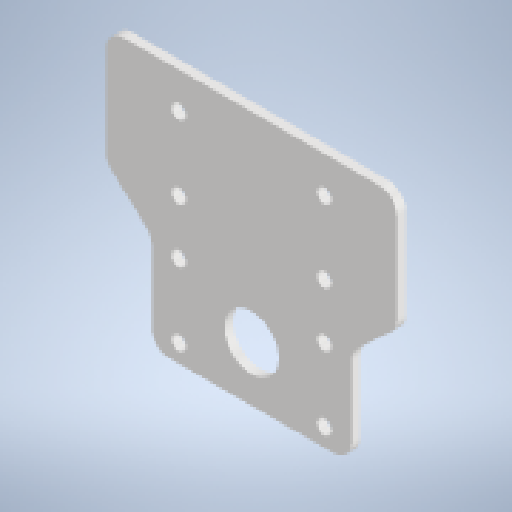
# Autodesk Inventor part: Dipper Plate (backplate)
Saved by Autodesk Inventor 2023 (Build 270158000, 158)
## iProperties
Created: 2023-03-02
Part Number: Dipper Plate (backplate)
Material: Generic
Document SubType Name: Modeling
Designer: Gabriel - T3 CAD
Density: 1 g/cm^3
Appearance: Default
Author: Gabriel - T3 CAD
Autodesk Inventor part; units mm, degrees
ref_plane "YZ Plane" through (0, 0, 0) normal (1, 0, 0) x (0, 1, 0)
ref_plane "XZ Plane" through (0, 0, 0) normal (0, 1, 0) x (-1, 0, 0)
ref_plane "XY Plane" through (0, 0, 0) normal (0, 0, 1) x (1, 0, 0)
sketch "Sketch1" plane through (0, 0, 0) normal (0, 0, 1) x (1, 0, 0)
  line L0 (0, 0) -> (-101.6, 0)
  line L1 (-101.6, 50.677) -> (-101.6, 95.25)
  line L2 (-101.6, 101.6) -> (-6.35, 101.6)
  line L3 (0, 95.25) -> (0, 50.677)
  circle A0 centre (-76.2, 88.9) radius 2.5797
  circle A1 centre (-76.2, 63.5) radius 2.5797
  circle A2 centre (-25.4, 88.9) radius 2.5797
  circle A3 centre (-25.4, 63.5) radius 2.5797
  circle A4 centre (-50.8, 19.05) radius 9.525
  circle A5 centre (-76.2, 31.75) radius 2.5797
  circle A6 centre (-76.2, 6.35) radius 2.5797
  circle A7 centre (-25.4, 31.75) radius 2.5797
  circle A8 centre (-25.4, 6.35) radius 2.5797
  line L4 (-85.725, 31.873) -> (-85.725, 6.35)
  line L5 (-85.725, 0) -> (-22.225, 0)
  line L6 (-15.875, 6.35) -> (-15.875, 31.873)
  arc A9 (0, 95.25) -> (-6.35, 101.6) centre (-6.35, 95.25) ccw
  line L7 (0, 0) -> (-79.375, 0)
  line L8 (-101.6, 50.677) -> (-101.6, 101.6)
  line L9 (-95.25, 101.6) -> (0, 101.6)
  line L10 (0, 101.6) -> (0, 50.677)
  arc A10 (-95.25, 101.6) -> (-101.6, 95.25) centre (-95.25, 95.25) ccw
  arc A11 (-22.225, 0) -> (-15.875, 6.35) centre (-22.225, 6.35) ccw
  arc A12 (-85.725, 6.35) -> (-79.375, 0) centre (-79.375, 6.35) ccw
  line L11 (-85.725, 47.625) -> (-101.6, 47.625)
  line L12 (-101.6, 47.625) -> (-101.6, 34.925)
  line L13 (-101.6, 34.925) -> (-85.725, 34.925)
  line L14 (-85.725, 34.925) -> (-85.725, 47.625)
  line L15 (-15.875, 47.625) -> (0, 47.625)
  line L16 (0, 47.625) -> (0, 34.925)
  line L17 (0, 34.925) -> (-15.875, 34.925)
  line L18 (-15.875, 34.925) -> (-15.875, 47.625)
  line L19 (-13.4918, 36.8315) -> (-2.3832, 45.7185)
  line L20 (-88.1082, 36.8315) -> (-99.2168, 45.7185)
  arc A13 (-2.3832, 45.7185) -> (0, 50.677) centre (-6.35, 50.677) ccw
  arc A14 (-13.4918, 36.8315) -> (-15.875, 31.873) centre (-9.525, 31.873) ccw
  arc A15 (-101.6, 50.677) -> (-99.2168, 45.7185) centre (-95.25, 50.677) ccw
  arc A16 (-85.725, 31.873) -> (-88.1082, 36.8315) centre (-92.075, 31.873) ccw
  point P0 (-15.875, 0)
  point P1 (-6.35, 101.6)
  point P2 (0, 95.25)
  point P3 (-101.6, 95.25)
  point P4 (-22.225, 0)
  point P5 (-79.375, 0)
  point P6 (-79.375, 0)
  point P7 (-85.725, 41.275)
  point P8 (-15.875, 41.275)
  dimension "d0" = 101.6
  dimension "d1" = 101.6
  dimension "d4" = 25.4
  dimension "d7" = 50.8
  dimension "d12" = 5.1594
  dimension "d13" = 19.05
  dimension "d14" = 5.1594
  dimension "d17" = 25.4
  dimension "d20" = 50.8
  dimension "d23" = 25.4
  dimension "d24" = 6.35
  dimension "d26" = 50.8
  dimension "d29" = 69.85
  dimension "d32" = 12.7
  dimension "d39" = 6.35
  dimension "d40" = 101.6
  dimension "d41" = 101.6
  dimension "d42" = 6.35
  dimension "d43" = 12.7
  dimension "d44" = 25.4
  dimension "d45" = 6.35
  dimension "d46" = 57.15
  dimension "d47" = 15.875
  dimension "d48" = 41.275
  dimension "d49" = 12.7
  dimension "d50" = 6.35
  constraints: 42 end point, 18 point on line, 17 centre point, 16 point on circle, 16 tangent, 9 parallel, 6 horizontal, 4 equal radius, 4 perpendicular, 3 equal length, 2 midpoint, 2 vertical, 12 other
  measures "d0" distance of L2.start point (0, 101.6)
  measures "d1" distance of L0.end L2.start
  measures "d4" distance of A0.centre A1.centre
  measures "d7" distance of A0.centre A2.centre
  measures "d12" diameter of A0
  measures "d13" diameter of A4
  measures "d14" diameter of A5
  measures "d17" distance of A5.centre A6.centre
  measures "d20" distance of A5.centre A7.centre
  measures "d23" distance from line of L1 A5.centre
  measures "d24" distance from line of L0 A6.centre
  measures "d26" distance from line of L1 A4.centre
  measures "d29" distance between parallel lines of L6 L4
  measures "d32" vertical distance of A6.centre A4.centre
  measures "d39" radius of A9
  measures "d40" distance of L2.start L9.end
  measures "d41" distance of point (-101.6, 0) L2.start
  measures "d42" radius of A10
  measures "d43" distance from line of L2 A0.centre
  measures "d44" distance from line of L1 A0.centre
  measures "d45" radius of A11
  measures "d46" distance of L7.end L5.end
  measures "d47" distance between parallel lines of L10 L6
  measures "d48" distance from line of point (-15.875, 41.275) L7
  measures "d49" distance between parallel lines of L15 L17
  measures "d50" radius of A13
extrude "Extrusion1" add sketch "Sketch1" along normal blind 3.175 contours L0 A12 L4 A16 L13 L14 L11 A15 L1 A10 L2 A9 L3 A13 L15 L18 L17 A14 L6 A11 | L17 L18 L15 A13 L19 A14 | A16 L20 A15 L11 L14 L13
body "Solid1"
